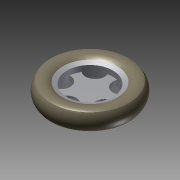
# Autodesk Inventor part: wheel
Saved by Autodesk Inventor 2012 (Build 160160000, 160)
## iProperties
Created: 2012-03-07
Part Number: wheel
Material: Default
Document SubType Name: Modeling
Designer: esv
Density: 0.813312 g/cm^3
Mass: 3526.68 g
Surface Area: 2513.34 cm^2
Volume: 4336.2 cm^3
Author: esv
Autodesk Inventor part; units mm, degrees
ref_plane "YZ Plane" through (0, 0, 0) normal (1, 0, 0) x (0, 1, 0)
ref_plane "XZ Plane" through (0, 0, 0) normal (0, 1, 0) x (-1, 0, 0)
ref_plane "XY Plane" through (0, 0, 0) normal (0, 0, 1) x (1, 0, 0)
sketch "Sketch1" plane through (0, 0, 0) normal (0, 0, 1) x (1, 0, 0)
  line L0 (0, 0) -> (0, 24.1958)
  arc A0 (158.75, -33.3375) -> (158.75, 33.3375) centre (121.3445, 0) ccw
  line L1 (171.45, -6.5142) -> (171.45, 28.0751)
  line L2 (93.6625, 22.225) -> (93.6625, -22.225)
  line L3 (93.6625, -22.225) -> (111.125, -28.575)
  line L4 (93.6625, 22.225) -> (111.125, 28.575)
  arc A1 (158.75, 33.3375) -> (111.125, 28.575) centre (139.3963, -13.6313) ccw
  arc A2 (111.125, -28.575) -> (158.75, -33.3375) centre (139.3963, 13.6313) ccw
  point P0 (93.6625, 0)
  dimension "d0" = 171.45
  dimension "d1" = 66.675
  dimension "d2" = 12.7
  dimension "d3" = 93.6625
  dimension "d4" = 111.125
  dimension "d5" = 44.45
  dimension "d6" = 57.15
  dimension "d7" = 50.8
  constraints: 10 end point, 6 point on circle, 3 centre point, 3 vertical alignment, 2 horizontal alignment, 2 parallel, 1 equal length, 1 midpoint, 1 tangent, 1 vertical
  measures "d0" distance between parallel lines of L0 L1
  measures "d1" distance of A0.end A0.start
  measures "d2" distance from line of L1 A0.end
  measures "d3" distance between parallel lines of L0 L2
  measures "d4" distance from line of L0 L4.end
  measures "d5" distance of L2.start L2.end
  measures "d6" distance of L3.end L4.end
  measures "d7" radius of A1
revolve "Revolution1" add sketch "Sketch1" angle 360 about axis through (0, 0, 0) along (0, 1, 0)
sketch "Sketch2" plane through (0, 0, 0) normal (0, 1, 0) x (-1, 0, 0)
  arc A0 (-38.1, 87.2981) -> (38.1, 87.2981) centre (0, 94.6626) ccw
  arc A1 (-94.7989, -9.2587) -> (-71.2518, 63.2118) centre (-90.0295, 29.2524) ccw
  arc A2 (-20.489, -93.0202) -> (-82.1361, -48.231) centre (-55.6413, -76.5837) ccw
  arc A3 (82.1361, -48.231) -> (20.489, -93.0202) centre (55.6413, -76.5837) ccw
  arc A4 (71.2518, 63.2118) -> (94.7989, -9.2587) centre (90.0295, 29.2524) ccw
  arc A5 (82.1361, -48.231) -> (94.7989, -9.2587) centre (0, 0) ccw
  arc A6 (-20.489, -93.0202) -> (20.489, -93.0202) centre (0, 0) ccw
  arc A7 (71.2518, 63.2118) -> (-71.2518, 63.2118) centre (0, 0) ccw
  arc A8 (-94.7989, -9.2587) -> (-82.1361, -48.231) centre (0, 0) ccw
  dimension "d10" = 76.2
  dimension "d13" = 360
  constraints: 20 point on circle, 9 centre point, 1 coincident, 1 vertical alignment, 21 other
  measures "d10" distance of A0.end A0.start
extrude "Extrusion1" add sketch "Sketch2" against normal blind 19.05 contours A0 A7 A4 A5 A3 A6 A2 A8 A1
body "Solid1"
